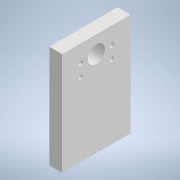
# Autodesk Inventor part: X Axis Plate
Saved by Autodesk Inventor 2022.3 (Build 263350000, 350)
## iProperties
Created: 2022-06-12
Part Number: X Axis Plate
Material: Generic
Document SubType Name: Modeling
Designer: Robert Nies
Density: 1 g/cm^3
Appearance: Default
Author: Robert Nies
Autodesk Inventor part; units mm, degrees
ref_plane "YZ Plane" through (0, 0, 0) normal (1, 0, 0) x (0, 1, 0)
ref_plane "XZ Plane" through (0, 0, 0) normal (0, 1, 0) x (-1, 0, 0)
ref_plane "XY Plane" through (0, 0, 0) normal (0, 0, 1) x (1, 0, 0)
sketch "Sketch1" plane through (0, 0, 0) normal (1, 0, 0) x (0, 1, 0)
  line L0 (0, 0) -> (114.3, 0)
  line L1 (114.3, 0) -> (114.3, -101.6)
  line L2 (114.3, -101.6) -> (0, -101.6)
  line L3 (0, -101.6) -> (0, 0)
  dimension "d0" = 114.3
  dimension "d1" = 101.6
  constraints: 8 end point, 2 parallel, 1 horizontal, 1 perpendicular
  measures "d0" distance of L1.end L2.end
  measures "d1" distance of L0.end L1.end
extrude "Extrusion1" add sketch "Sketch1" along normal blind 19.05
sketch "Sketch2" plane through (19.05, 0, 0) normal (1, 0, 0) x (0, 0, -1)
  circle A0 centre (27.8, 88.9) radius 3.2499
  circle A1 centre (73.8, 88.9) radius 3.2499
  circle A2 centre (73.8, 70.9) radius 3.2499
  circle A3 centre (27.8, 70.9) radius 3.2499
  line L0 (27.8, 88.9) -> (27.8, 70.9)
  line L1 (27.8, 88.9) -> (73.8, 88.9)
  line L2 (27.8, 70.9) -> (73.8, 70.9)
  line L3 (73.8, 70.9) -> (73.8, 88.9)
  line L4 (0, 114.3) -> (0, 0) projected
  line L5 (101.6, 0) -> (101.6, 114.3) projected
  line L6 (101.6, 114.3) -> (0, 114.3) projected
  dimension "d4" = 6.4999
  dimension "d5" = 6.4999
  dimension "d6" = 6.4999
  dimension "d7" = 6.4999
  dimension "d8" = 46
  dimension "d9" = 18
  dimension "d10" = 27.8
  dimension "d11" = 101.6
  dimension "d12" = 25.4
  constraints: 8 end point, 4 centre point, 2 horizontal, 2 vertical
  measures "d4" diameter of A0
  measures "d5" diameter of A1
  measures "d6" diameter of A2
  measures "d7" diameter of A3
  measures "d8" distance of L1.end L0.start
  measures "d9" distance of L0.end L0.start
  measures "d10" distance from line of L4 L0.start
  measures "d11" distance between parallel lines of L5 L4
  measures "d12" distance from line of L6 L0.start
extrude "Extrusion2" cut sketch "Sketch2" against normal blind 19.05 contours L1 L0 A0 | A0 L0 L1 | L1 L3 A1 | A1 L3 L1 | L0 L2 A3 | A3 L2 L0 | L3 L2 A2 | A2 L2 L3
sketch "Sketch4" plane through (0, 0, 0) normal (-1, 0, 0) x (0, 0, 1)
  circle A0 centre (-50.8, 88.9) radius 12.7
  line L0 (-101.6, 114.3) -> (0, 114.3) projected
  circle A1 centre (-73.8, 88.9) radius 3.2499 projected
  circle A2 centre (-27.8, 88.9) radius 3.2499 projected
  line L1 (-73.8, 88.9) -> (-27.8, 88.9)
  point P0 (0, 0)
  dimension "d15" = 25.4
  constraints: 2 end point, 1 centre point, 1 horizontal, 1 midpoint
  measures "d15" diameter of A0
extrude "Extrusion3" cut sketch "Sketch4" against normal blind 19.05 contours L1 A0 | A0 L1
equation "\"d10\" = -0.5 * d8 + 0.5 * d11"
body "Solid1"
